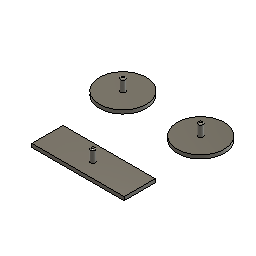
Insert_Blanks_OkoLabs (Autodesk Fusion 360 design; units mm, degrees)
Autodesk Fusion 360 part; units mm, degrees
sketch "Sketch1" plane through (0, 0, 0) normal (0, 1, 0) x (1, 0, 0)
  circle A0 centre (0, 0) radius 19.5
  dimension "d1" = 39
  constraint coincident A0.centre origin
  measures "d1" diameter of A0
extrude "Extrude1" add sketch "Sketch1" along normal blind 3 makes body 1
sketch "Sketch2" plane through (0, 0, 0) normal (0, 1, 0) x (1, 0, 0)
  circle A0 centre (0, 0) radius 2
  dimension "d4" = 4
  constraint coincident A0.centre origin
  measures "d4" diameter of A0
extrude "Extrude2" add sketch "Sketch2" along normal blind 13 bodies 1
fillet "Fillet1" radius 1 1 edges at (-1.8647, 13, 0.7232) on bodies 1
sketch "Sketch3" plane through (0, 0, 0) normal (0, 1, 0) x (1, 0, 0)
  circle A0 centre (65, 0) radius 19.5
  dimension "d8" = 39
  measures "d8" diameter of A0
extrude "Extrude3" add sketch "Sketch3" along normal blind 3 separate body makes body 2
sketch "Sketch4" plane through (0, 0, 0) normal (0, 1, 0) x (1, 0, 0)
  circle A0 centre (65, 0) radius 2
  dimension "d11" = 4
  measures "d11" diameter of A0
extrude "Extrude4" add sketch "Sketch4" along normal blind 13 bodies 2
fillet "Fillet2" radius 1 1 edges at (63.1353, 13, 0.7232) on bodies 2
sketch "Sketch5" plane through (0, 0, 0) normal (0, 1, 0) x (1, 0, 0)
  line L0 (0, -50) -> (77, -50)
  line L1 (77, -50) -> (77, -76)
  line L2 (77, -76) -> (0, -76)
  line L3 (0, -76) -> (0, -50)
  dimension "d15" = 77
  dimension "d16" = 26
  constraint horizontal L0
  constraint vertical L1
  constraint horizontal L2
  constraint vertical L3
  measures "d15" distance of L0.start L0.end
  measures "d16" distance of L0.start L2.end
extrude "Extrude5" add sketch "Sketch5" along normal blind 3 separate body makes body 3
sketch "Sketch6" plane through (0, 0, 0) normal (0, 1, 0) x (1, 0, 0)
  circle A0 centre (38.5, -63.6937) radius 2
  dimension "d19" = 4
  measures "d19" diameter of A0
extrude "Extrude6" add sketch "Sketch6" along normal blind 13 bodies 3
fillet "Fillet3" radius 1 1 edges at (36.6353, 13, 64.4169) on bodies 3
